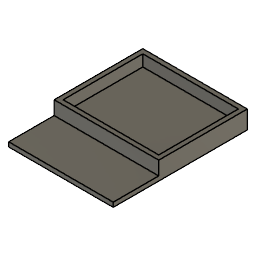
MotorController_Halterung (Autodesk Fusion 360 design; units mm, degrees)
Autodesk Fusion 360 part; units mm, degrees
box "Grundkörper Quader1" add length 39 width 46 height 2 placed x (0, -1, 0) y (1, 0, 0) z (0, 0, 1) at (0, 0, 0) makes body 1
box "Grundkörper Quader2" add length 39 width 46 height 5 placed x (0, -1, 0) y (1, 0, 0) z (0, 0, 1) at (0, 0, 2) separate body makes body 2
shell "Schale1" thickness 2 removed faces 2 at (30.6667, -13, 7) at (30.6667, -13, 2) on bodies 2
extrude "Extrusion1" add 1 faces at (30.6667, -39, 0.6667) along direction (0, -1, 0) blind 20 on bodies 1 bodies 1 2
extrude "Extrusion2" add 1 faces at (30, -13.6667, 2) along direction (0, 0, 1) blind 1 on bodies 1 bodies 1
extrude "Extrusion3" add 1 faces at (30, -0.6667, 7) along direction (0, 0, 1) blind 1 on bodies 1 bodies 1
